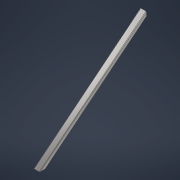
# Autodesk Inventor part: support_truss2
Saved by Autodesk Inventor 2021 (Build 250183000, 183)
## iProperties
Created: 2021-05-11
Part Number: support_truss2
Material: Steel, Galvanized
Document SubType Name: Modeling
Designer: Watchdog
Density: 7.85 g/cm^3
Appearance: Galvanized
Author: Watchdog
Autodesk Inventor part; units mm, degrees
ref_plane "YZ Plane" through (0, 0, 0) normal (1, 0, 0) x (0, 1, 0)
ref_plane "XZ Plane" through (0, 0, 0) normal (0, 1, 0) x (-1, 0, 0)
sketch "profile" plane through (0, 0, 0) normal (0, 1, 0) x (-1, 0, 0)
  line L0 (12.5, 12.5) -> (-12.5, 12.5)
  line L1 (-12.5, 12.5) -> (-12.5, -12.5)
  line L2 (-12.5, -12.5) -> (12.5, -12.5)
  line L3 (12.5, -12.5) -> (12.5, 12.5)
  line L4 (-10, -10) -> (-10, 10)
  line L5 (-10, 10) -> (10, 10)
  line L6 (10, 10) -> (10, -10)
  line L7 (10, -10) -> (-10, -10)
  point P0 (0, 0)
  dimension "d0" = 12.5
  dimension "d1" = 25
  dimension "d2" = 25
  dimension "d3" = 12.5
  dimension "d6" = 2.5
  constraints: 16 end point, 4 parallel, 2 perpendicular, 1 horizontal, 3 other
  measures "d0" distance from line of point (0, 0) L0
  measures "d1" distance of L2.end L0.start
  measures "d2" distance of L0.start L0.end
  measures "d3" distance from line of point (0, 0) L3
  measures "d6" distance between parallel lines of L1 L4
sketch3d "3D Sketch1"
  line L0 (0, 0, 0) -> (0, 397.8712, -494.9758)
  dimension "d4" = 635.061
  dimension "d5" = 38.793
sweep "Sweep1" add profiles "profile" path "3D Sketch1"
fillet "Fillet1" radius 2 4 edges at (-12.5, 198.9356, -259.9879) (-12.5, 198.9356, -234.9879) (12.5, 198.9356, -234.9879) (12.5, 198.9356, -259.9879)
ref_plane "Work Plane2" through (-10.5, 351.8712, -507.4758) normal (0, 1, 0) x (1, 0, 0)
split "Split2" plane through (-10.5, 351.8712, -507.4758) removes the side toward (0, 1, 0)
ref_plane "Work Plane3" through (0, 351.8712, -425.249) normal (0, 0, 1) x (1, 0, 0)
split "Split3" plane through (0, 351.8712, -425.249) removes the side toward (0, 0, -1)
equation "\"d0\" = 0.5 * d1"
equation "\"d1\" = width"
equation "\"d2\" = d1"
equation "\"d3\" = 0.5 * d2"
equation "\"d6\" = t"
equation "\"d4\" = L"
equation "\"d5\" = angle"
equation "\"d9\" = filletRadius"
equation "\"L\" = 635.061"
equation "\"t\" = 2.5"
equation "\"filletRadius\" = 2"
equation "\"angle\" = 38.793deg"
equation "\"width\" = 25"
body "Solid1"
